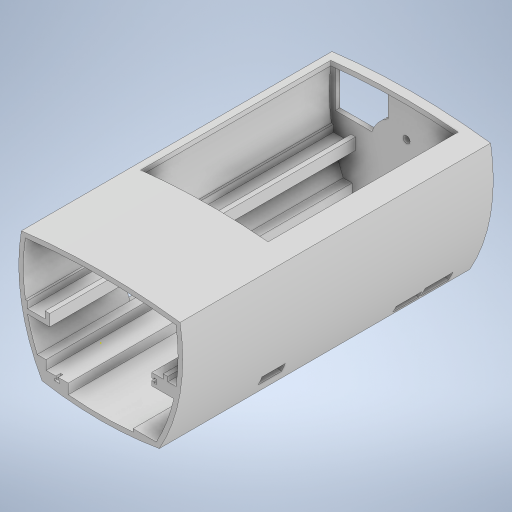
# Autodesk Inventor part: testingagain
Saved by Autodesk Inventor 2023 (Build 270158000, 158)
## iProperties
Created: 2022-11-19
Part Number: testingagain
Material: Generic
Document SubType Name: Modeling
Designer: jeron
Density: 1 g/cm^3
Appearance: Default
Author: jeron
Autodesk Inventor part; units mm, degrees
sketch "Sketch1" plane through (0, 0, 0) normal (0, 0, 1) x (1, 0, 0)
  line L0 (-32.5, 23) -> (32.5, 23)
  line L1 (32.5, 23) -> (32.5, 0)
  line L2 (-32.5, 0) -> (-32.5, 23)
  line L3 (-24, -18) -> (-24, 0)
  line L4 (24, -25) -> (24, -5)
  line L5 (0, -25) -> (24, -25)
  line L6 (0, -25) -> (-14, -25)
  line L7 (0, 23) -> (0, 25)
  line L8 (0, -25) -> (0, -27)
  arc A0 (-32.5, 23) -> (-24, -25) centre (42.3382, 11.5) ccw
  line L9 (-32.5, 0) -> (-31.5587, 0)
  line L10 (-24, 0) -> (-24, -5)
  line L11 (32.5, 0) -> (24, 0)
  line L12 (24, 0) -> (24, -5)
  line L13 (24, -5) -> (31.5587, -5)
  line L14 (24, -25) -> (15.6259, -25)
  line L15 (24, -25) -> (14, -25)
  line L16 (14, -25) -> (14, -26.3226)
  line L17 (-14, -25) -> (-14, -26.3226)
  arc A1 (32.5, 23) -> (-32.5, 23) centre (0, -240.0625) ccw
  arc A2 (24, -25) -> (32.5, 23) centre (-42.3382, 11.5) ccw
  arc A3 (-24, -25) -> (24, -25) centre (0, 118) ccw
  arc A4 (-34.2324, 24.7969) -> (-25.28, -26.8099) centre (42.3382, 11.5) ccw
  arc A5 (-25.28, -26.8099) -> (25.28, -26.8099) centre (0, 118) ccw
  arc A6 (25.28, -26.8099) -> (34.2324, 24.7969) centre (-42.3382, 11.5) ccw
  arc A7 (34.2324, 24.7969) -> (-34.2324, 24.7969) centre (0, -240.0625) ccw
  line L18 (-14, -25) -> (-14, -22)
  line L19 (-14, -22) -> (-25.5644, -22)
  line L20 (-24, -5) -> (-22, -5)
  line L21 (-22, -5) -> (-22, 0)
  line L22 (-31.5587, -5) -> (-31.5587, 0)
  line L23 (-32.5, 0) -> (-31.5587, 0)
  line L24 (-24, 0) -> (32.5, 0)
  line L25 (24, -5) -> (22, -5)
  line L26 (22, -5) -> (22, 0)
  line L27 (24, 0) -> (27, 0)
  line L28 (27, 0) -> (27, 2)
  line L29 (27, 2) -> (29, 2)
  line L30 (29, 2) -> (29, 0)
  line L31 (27, 0) -> (29, 0)
  line L32 (-25.5644, -22) -> (-23.5644, -22)
  line L33 (-23.5644, -22) -> (-23.5644, -18)
  line L34 (-23.5644, -18) -> (-27.3953, -18)
  line L35 (-24, -5) -> (-24, -3)
  line L36 (-24, -3) -> (-31.977, -3)
  line L37 (-24, -5) -> (-31.5587, -5)
  line L38 (0, 0) -> (0, -1.7837)
  point P0 (0, -28)
  point P1 (0, 26)
  point P2 (27, 0)
  point P3 (29, 0)
  point P4 (-31.5587, -3)
  point P5 (0, -29)
  point P6 (0, -27)
  point P7 (0, 27)
  point P8 (0, 25)
  dimension "d19" = 65
  dimension "d20" = 23
  dimension "d30" = 65
  dimension "d39" = 48
  dimension "d40" = 25
  dimension "d41" = 8.5
  dimension "d42" = 8.5
  dimension "d43" = 2
  dimension "d44" = 2
  dimension "d45" = 54
  dimension "d46" = 5
  dimension "d47" = 5
  dimension "d48" = 10
  dimension "d49" = 10
  dimension "d54" = 3
  dimension "d55" = 2
  dimension "d56" = 2
  dimension "d68" = 3
  dimension "d69" = 2
  dimension "d70" = 2
  dimension "d84" = 2
  dimension "d85" = 4
  dimension "d88" = 2
  dimension "d123" = 23
  dimension "d124" = 25
  dimension "d125" = 32.5
  dimension "d126" = 2
  dimension "d127" = 2
  constraints: 78 end point, 28 point on circle, 14 perpendicular, 12 point on line, 8 centre point, 7 horizontal, 4 collinear, 4 vertical, 1 midpoint, 1 parallel, 3 other
  measures "d19" distance of L0.start L0.end
  measures "d20" distance of L0.end L1.end
  measures "d30" distance of L1.end L2.start
  measures "d39" distance of L11.end L3.end
  measures "d40" distance of L4.start L11.end
  measures "d41" distance of L11.end L1.end
  measures "d42" distance of L2.start L3.end
  measures "d43" distance of L7.start L7.end
  measures "d44" distance of L5.start L8.end
  measures "d45" distance of point (0, -28) point (0, 26)
  measures "d46" distance of L3.end L10.end
  measures "d47" distance of L4.end L11.end
  measures "d48" distance of L14.start L15.end
  measures "d49" distance of L6.end A0.end
  measures "d54" distance of L6.end L18.end
  measures "d55" distance of L10.end L20.end
  measures "d56" distance of L4.end L25.end
  measures "d68" distance of L11.end L27.end
  measures "d69" distance of L27.end L28.end
  measures "d70" distance of L28.end L29.end
  measures "d84" distance of L19.end L32.end
  measures "d85" distance of L32.end L33.end
  measures "d88" distance of L10.end L35.end
  measures "d123" distance between parallel lines of L0 L24
  measures "d124" distance between parallel lines of L6 L24
  measures "d125" distance of L38.start L1.end
  measures "d126" distance of point (0, -29) point (0, -27)
  measures "d127" distance of point (0, 27) point (0, 25)
extrude "Extrusion3" add sketch "Sketch1" along normal blind 100 contours L9 L22 L36 A0 | L36 L22 A0 | A2 L13 L12 L11 | L3 L24 L21 L20 | L25 L26 L24 L12 | A3 L16 L5 | L19 L18 L17 A3 A0 | A7 A6 A5 A4
extrude "Extrusion4" add sketch "Sketch1" against normal blind 2 contours A1 L7 L0 | L0 L1 L11 L30 L29 L28 L24 L3 L36 L22 L9 L2 | L2 A0 | L7 A1 L0 | L9 L22 L36 A0 | A2 L1 | L36 L22 A0 | A2 L13 L12 L11 | L37 L3 L34 A0 | L22 L36 L3 L37 | L11 L28 L29 L30 | A2 L4 L13 | L34 L33 L19 A0 | L20 L21 L24 L26 L25 L4 L5 L6 L18 L19 L33 L34 L3 | L3 L24 L21 L20 | L25 L26 L24 L12 | A3 L16 L5 | L19 L18 L17 A3 A0 | A3 L8 L5 L16 | A3 L17 L6 L8 | A7 A6 A5 A4
ref_plane "Work Plane2" through (0, 27, 100) normal (0, 1, 0) x (-1, 0, 0)
sketch "Sketch2" plane through (0, 27, 100) normal (0, 1, 0) x (-1, 0, 0)
  line L0 (34.2324, -102) -> (34.2324, 0) projected
  line L1 (-34.2324, 0) -> (34.2324, 0) projected
  line L2 (-34.2324, -102) -> (-34.2324, 0) projected
  line L3 (34.2324, -102) -> (-34.2324, -102) projected
  line L4 (-34.2324, -102) -> (-27.2324, -102)
  line L5 (-27.2324, -102) -> (30.7676, -102)
  line L6 (30.7676, -102) -> (34.2324, -102)
  line L7 (34.2324, 0) -> (-34.2324, 0)
  line L8 (-27.2373, 0) -> (30.7627, 0)
  line L9 (30.7627, 0) -> (34.2324, 0)
  line L10 (-34.2324, -100) -> (-24.2324, -100)
  line L11 (-24.2324, -98) -> (30.7676, -98)
  line L12 (25.5644, -100) -> (31.5587, -100) projected
  line L13 (34.2324, -100) -> (30.7578, -100)
  line L14 (-24.2324, -98) -> (-24.2324, -16)
  line L15 (-25.28, 0) -> (-25.28, -102) projected
  line L16 (-24.2324, -98) -> (57.7676, -98) construction
  line L17 (25.5644, -100) -> (25.5644, 0) projected
  line L18 (31.5587, -100) -> (31.5587, 0) projected
  line L19 (-24.2324, -16) -> (30.7676, -16)
  line L20 (-24.2373, -18) -> (-24.2373, -16)
  line L21 (30.7676, -98) -> (30.7676, -16)
  point P0 (0, -100)
  point P1 (25.5644, -18)
  point P2 (31.5587, -18)
  point P3 (25.5644, -16)
  point P4 (-34.2324, -51)
  point P5 (25.5644, -98)
  dimension "d61" = 7
  dimension "d62" = 58
  dimension "d63" = 3.4649
  dimension "d64" = 82
  dimension "d65" = 90
  dimension "d73" = 2
  dimension "d74" = 10
  constraints: 26 end point, 8 point on line, 3 horizontal, 2 perpendicular, 1 collinear, 1 midpoint, 1 parallel, 1 vertical, 3 other
  measures "d61" distance of L2.start L4.end
  measures "d62" distance of L4.end L5.end
  measures "d63" distance of L0.start L5.end
  measures "d64" distance of L14.start L14.end
  measures "d65" angle of L16 L14
  measures "d73" distance of L20.start L20.end
  measures "d74" distance from line of L14 point (-34.232, -51)
extrude "Extrusion5" cut sketch "Sketch2" against normal up to surface contours L17 L19 L21 L11 | L11 L14 L19 L17
sketch "Sketch3" plane through (0, 0, 0) normal (0, 0, 1) x (1, 0, 0)
  point P0 (0, 0)
ref_plane "Work Plane4" through (34.2348, -1.7834, -2) normal (0.9852847, -0.1709212, 0) x (0.1709212, 0.9852847, 0)
sketch "Sketch5" plane through (34.2348, -1.7834, -2) normal (0.9852847, -0.1709212, 0) x (0.1709212, 0.9852847, 0)
  line L0 (-24.6243, 2) -> (-24.6243, 102) projected
  line L1 (-24.6243, 2) -> (-24.6243, 10)
  line L2 (-24.6243, 10) -> (-20.6243, 10)
  line L3 (-20.6243, 10) -> (-20.6243, 22)
  line L4 (-20.6243, 22) -> (-24.6243, 22)
  line L5 (-24.6243, 22) -> (-24.6243, 23)
  line L6 (-24.6243, 23) -> (-21.6243, 23)
  line L7 (-21.6243, 23) -> (-21.6243, 34)
  line L8 (-21.6243, 34) -> (-24.6243, 34)
  line L9 (-24.6243, 2) -> (-24.6243, 84)
  line L10 (-24.6243, 84) -> (-16.6243, 84)
  line L11 (-16.6243, 84) -> (-16.6243, 94)
  line L12 (-16.6243, 94) -> (-24.6243, 94)
  line L13 (-24.6243, 84) -> (-20.6243, 84)
  line L14 (-20.6243, 84) -> (-20.6243, 94)
  point P0 (-4.0943, 2)
  dimension "d76" = 8
  dimension "d77" = 4
  dimension "d78" = 12
  dimension "d79" = 1
  dimension "d80" = 3
  dimension "d81" = 11
  dimension "d91" = 82
  dimension "d92" = 8
  dimension "d93" = 10
  dimension "d94" = 4
  constraints: 28 end point, 8 perpendicular, 6 point on line, 2 midpoint, 1 vertical
  measures "d76" distance of L0.start L1.end
  measures "d77" distance of L1.end L2.end
  measures "d78" distance of L2.end L3.end
  measures "d79" distance of L4.end L5.end
  measures "d80" distance of L5.end L6.end
  measures "d81" distance of L6.end L7.end
  measures "d91" distance of L0.start L9.end
  measures "d92" distance of L9.end L10.end
  measures "d93" distance of L10.end L11.end
  measures "d94" distance of L9.end L13.end
extrude "Extrusion7" cut sketch "Sketch5" against normal blind 10 contours L0 L4 L3 L2 | L0 L8 L7 L6 | L14 L12 L11 L10
extrude "Extrusion8" add sketch "Sketch1" along normal up to surface (100 mm away) contours L11 L28 L29 L30 | L34 L33 L19 A0
extrude "Extrusion9" add sketch "Sketch1" along normal up to surface (100 mm away) contours L22 L36 L3 L37
ref_plane "Work Plane5" through (-34.2348, -1.7834, 100) normal (-0.9852847, -0.1709212, 0) x (0.1709212, -0.9852847, 0)
sketch "Sketch6" plane through (-34.2348, -1.7834, 100) normal (-0.9852847, -0.1709212, 0) x (0.1709212, -0.9852847, 0)
  line L0 (17.147, 0) -> (17.147, -100) projected
  line L1 (17.147, -100) -> (17.147, -18)
  line L2 (17.147, -18) -> (13.147, -18)
  line L3 (13.147, -18) -> (13.147, -8)
  line L4 (13.147, -8) -> (17.147, -8)
  point P0 (4.0943, -100)
  dimension "d95" = 82
  dimension "d96" = 4
  dimension "d97" = 10
  constraints: 8 end point, 3 perpendicular, 2 point on line
  measures "d95" distance of L0.end L1.end
  measures "d96" distance of L1.end L2.end
  measures "d97" distance of L2.end L3.end
extrude "Extrusion10" cut sketch "Sketch6" against normal blind 10
ref_plane "Work Plane6" through (34.2324, 24.7969, 100) normal (0, 0, 1) x (1, 0, 0)
sketch "Sketch7" plane through (34.2324, 24.7969, 100) normal (0, 0, 1) x (1, 0, 0)
  arc A0 (0, 0) -> (-68.4649, 0) centre (-34.2324, -264.8594) ccw projected
  arc A1 (-68.4649, 0) -> (-59.5124, -51.6069) centre (8.1058, -13.2969) ccw projected
  arc A2 (-66.7324, -1.7969) -> (-66.7324, -24.7969) centre (8.1058, -13.2969) ccw projected
  arc A3 (-1.7324, -1.7969) -> (-66.7324, -1.7969) centre (-34.2324, -264.8594) ccw projected
  arc A4 (-8.9524, -51.6069) -> (0, 0) centre (-76.5707, -13.2969) ccw projected
  arc A5 (-1.7324, -24.7969) -> (-1.7324, -1.7969) centre (-76.5707, -13.2969) ccw projected
  line L0 (-1.7324, -24.7969) -> (-5.2324, -24.7969) projected
  line L1 (-5.2324, -22.7969) -> (-5.2324, -24.7969) projected
  line L2 (-7.2324, -22.7969) -> (-5.2324, -22.7969) projected
  line L3 (-7.2324, -24.7969) -> (-7.2324, -22.7969) projected
  line L4 (-7.2324, -24.7969) -> (-12.2324, -24.7969) projected
  line L5 (-12.2324, -24.7969) -> (-12.2324, -29.7969) projected
  line L6 (-12.2324, -29.7969) -> (-2.6737, -29.7969) projected
  arc A6 (-10.2324, -49.7969) -> (-2.6737, -29.7969) centre (-76.5707, -13.2969) ccw projected
  line L7 (-65.7912, -24.7969) -> (-66.7324, -24.7969) projected
  line L8 (-65.7912, -27.7969) -> (-65.7912, -24.7969) projected
  line L9 (-65.7912, -27.7969) -> (-58.2324, -27.7969) projected
  line L10 (-58.2324, -24.7969) -> (-58.2324, -27.7969) projected
  line L11 (-56.2324, -24.7969) -> (-58.2324, -24.7969) projected
  line L12 (-56.2324, -29.7969) -> (-56.2324, -24.7969) projected
  line L13 (-56.2324, -29.7969) -> (-65.7912, -29.7969) projected
  arc A7 (-65.7912, -29.7969) -> (-61.6277, -42.7969) centre (8.1058, -13.2969) ccw projected
  line L14 (-61.6277, -42.7969) -> (-57.7968, -42.7969) projected
  line L15 (-57.7968, -42.7969) -> (-57.7968, -46.7969) projected
  line L16 (-48.2324, -46.7969) -> (-57.7968, -46.7969) projected
  line L17 (-48.2324, -51.1195) -> (-48.2324, -46.7969) projected
  arc A8 (-48.2324, -51.1195) -> (-20.2324, -51.1195) centre (-34.2324, 93.2031) ccw projected
  line L18 (-20.2324, -49.7969) -> (-20.2324, -51.1195) projected
  line L19 (-10.2324, -49.7969) -> (-20.2324, -49.7969) projected
  arc A9 (-59.5124, -51.6069) -> (-8.9524, -51.6069) centre (-34.2324, 93.2031) ccw projected
  point P0 (-34.2324, -24.7969)
extrude "Extrusion11" add sketch "Sketch7" along normal blind 32
sketch "Sketch8" plane through (0, 0, -2) normal (0, 0, -1) x (-1, 0, 0)
  circle A0 centre (0, 0) radius 16
  arc A1 (30.7676, 23.2082) -> (-24.2324, 23.89) centre (0, -240.0625) ccw projected
  line L0 (30.7676, 23.2082) -> (7.9501, 23.2082)
  line L1 (7.9501, 23.2082) -> (7.9501, 13.8851)
  line L2 (15.0321, 5.4805) -> (30.7676, 5.4805)
  line L3 (30.7676, 5.4805) -> (30.7676, 23.2082)
  circle A2 centre (0, 10) radius 1.5
  circle A3 centre (0, -10) radius 1.5
  dimension "d102" = 32
  dimension "d104" = 3
  dimension "d106" = 3
  dimension "d121" = 10
  dimension "d122" = 10
  dimension "d128" = 7.9501
  dimension "d129" = 13.8851
  dimension "d130" = 22.8175
  dimension "d131" = 17.7278
  constraints: 8 end point, 3 centre point, 2 horizontal, 2 perpendicular, 2 point on circle, 1 coincident
  measures "d102" diameter of A0
  measures "d104" diameter of A2
  measures "d106" diameter of A3
  measures "d121" distance of point (0, 0) A2.centre
  measures "d122" distance of point (0, 0) A3.centre
  measures "d128" horizontal distance of point (0, 0) L1.end
  measures "d129" vertical distance of point (0, 0) L1.end
  measures "d130" distance of L0.end L0.start
  measures "d131" distance of L2.end L0.start
extrude "Extrusion12" cut sketch "Sketch8" against normal up to surface (2 mm away) contours A0 L1 L0 L3 L2 | A2 | A3
sketch "Sketch9" plane through (34.2324, 24.7969, 132) normal (0, 0, 1) x (1, 0, 0)
  point P0 (-34.2324, -24.7969)
sketch "Sketch10" plane through (34.2324, 24.7969, 132) normal (0, 0, 1) x (1, 0, 0)
  line L0 (-12.2324, -24.7969) -> (-12.2324, -29.7969) projected
  line L1 (-10.2373, -27.302) -> (-10.2373, -26.302)
  line L2 (-10.2373, -27.302) -> (-10.2373, -28.302)
  line L3 (-10.2373, -28.302) -> (-11.2373, -28.302)
  line L4 (-11.2373, -26.302) -> (-10.2373, -26.302)
  line L5 (-11.2373, -26.7969) -> (-12.2324, -26.7969)
  line L6 (-11.2373, -27.7969) -> (-12.2324, -27.7969)
  line L7 (-11.2373, -28.302) -> (-11.2373, -27.7969)
  line L8 (-11.2373, -26.7969) -> (-11.2373, -26.302)
  line L9 (-48.2324, -46.7969) -> (-57.7968, -46.7969) projected
  line L10 (-52.5195, -47.802) -> (-52.0195, -47.802)
  line L11 (-52.0195, -47.802) -> (-52.0195, -48.802)
  line L12 (-52.0195, -48.802) -> (-54.0195, -48.802)
  line L13 (-54.0195, -48.802) -> (-54.0195, -47.802)
  line L14 (-52.5195, -47.802) -> (-52.5195, -46.7969)
  line L15 (-53.5195, -47.802) -> (-53.5195, -46.7969)
  line L16 (-54.0195, -47.802) -> (-53.5195, -47.802)
  line L17 (-53.5195, -46.7969) -> (-52.5195, -46.7969)
  line L18 (-12.2324, -26.7969) -> (-12.2324, -27.7969)
  point P0 (-34.2324, -24.7969)
  dimension "d110" = 1
  dimension "d111" = 1
  dimension "d112" = 1
  dimension "d113" = 2
  dimension "d116" = 1
  dimension "d117" = 2
  dimension "d118" = 1
  constraints: 34 end point, 9 perpendicular, 4 point on line, 1 collinear, 1 horizontal, 1 vertical
  measures "d110" distance of L1.start L1.end
  measures "d111" distance of L1.start L2.end
  measures "d112" distance of L2.end L3.end
  measures "d113" distance of L3.end L4.start
  measures "d116" distance of L10.end L11.end
  measures "d117" distance of L11.end L12.end
  measures "d118" distance of L12.end L13.end
extrude "Extrusion13" cut sketch "Sketch10" against normal blind 2
body "Solid2"
